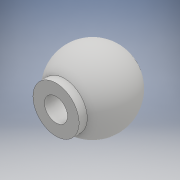
# Autodesk Inventor part: ballJoint
Saved by Autodesk Inventor 2018 (Build 220112000, 112)
## iProperties
Created: 2020-03-25
Part Number: ballJoint
Material: Generic
Document SubType Name: Modeling
Designer: technik
Density: 1 g/cm^3
Appearance: Default
Author: technik
Autodesk Inventor part; units mm, degrees
ref_plane "YZ Plane" through (0, 0, 0) normal (1, 0, 0) x (0, 1, 0)
ref_plane "XZ Plane" through (0, 0, 0) normal (0, 1, 0) x (-1, 0, 0)
ref_plane "XY Plane" through (0, 0, 0) normal (0, 0, 1) x (1, 0, 0)
sketch "Sketch1" plane through (0, 0, 0) normal (0, 0, 1) x (1, 0, 0)
  arc A0 (0, 2.375) -> (-1.5, -1.8414) centre (0, 0) ccw
  line L0 (0, 2.375) -> (0, -2.375)
  line L1 (0, -2.375) -> (-1.5, -2.375)
  line L2 (-1.5, -2.375) -> (-1.5, -1.8414)
  dimension "d0" = 4.75
  dimension "d1" = 1.5
  constraints: 6 end point, 2 perpendicular, 2 point on circle, 1 centre point, 1 coincident, 1 vertical
  measures "d0" diameter of A0
  measures "d1" distance of L0.end L1.end
revolve "Revolution1" add sketch "Sketch1" angle 360 about axis through (0, 2.375, 0) along (0, -1, 0)
sketch "Sketch2" plane through (0, -2.375, 0) normal (0, -1, 0) x (1, 0, 0)
  circle A0 centre (0, 0) radius 0.75
  dimension "d3" = 1.5
  constraints: 1 centre point, 1 coincident
  measures "d3" diameter of A0
extrude "Extrusion1" cut sketch "Sketch2" against normal blind 10
chamfer "Chamfer1" distance 0.5 angle 45 2 edges at (0, 2.2535, -0.75) (0, 2.2535, 0.75)
body "Solid1"
